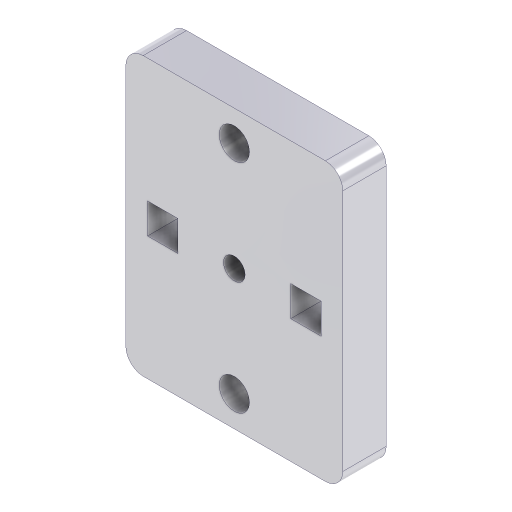
# Autodesk Inventor part: I Rückwand Adapter
Saved by Autodesk Inventor 2023 (Build 270158000, 158)
## iProperties
Created: 2022-09-18
Part Number: I Rückwand Adapter
Material: PBT-Kunststoff
Document SubType Name: Modeling
Designer: musati
Density: 1.31 g/cm^3
Appearance: Opal
Author: musati
Autodesk Inventor part; units mm, degrees
ref_plane "YZ Plane" through (0, 0, 0) normal (1, 0, 0) x (0, 1, 0)
ref_plane "XZ Plane" through (0, 0, 0) normal (0, 1, 0) x (-1, 0, 0)
ref_plane "XY Plane" through (0, 0, 0) normal (0, 0, 1) x (1, 0, 0)
sketch "Skizze1" plane through (0, 0, 0) normal (0, 0, 1) x (1, 0, 0)
  line L0 (-18.0799, 0) -> (18.0799, 0) projected
  line L1 (0, -22.9799) -> (0, 22.9799) projected
  line L2 (-10.5, -16) -> (10.5, -16)
  line L3 (12.5, -14) -> (12.5, 14)
  line L4 (10.5, 16) -> (-10.5, 16)
  line L5 (-12.5, 14) -> (-12.5, -14)
  line L6 (-12.5, -16) -> (12.5, 16) construction
  line L7 (12.5, -16) -> (-12.5, 16) construction
  arc A0 (-10.5, 16) -> (-12.5, 14) centre (-10.5, 14) ccw
  arc A1 (-12.5, -14) -> (-10.5, -16) centre (-10.5, -14) ccw
  arc A2 (10.5, -16) -> (12.5, -14) centre (10.5, -14) ccw
  arc A3 (12.5, 14) -> (10.5, 16) centre (10.5, 14) ccw
  point P0 (0, 0)
  dimension "d0" = 25
  dimension "d1" = 32
  dimension "d2" = 2
  constraints: 12 end point, 8 point on circle, 8 point on line, 8 tangent, 4 centre point, 3 equal radius, 2 midpoint, 2 parallel, 1 horizontal, 1 perpendicular
  measures "d0" distance of L7.end L6.end
  measures "d1" distance of L6.end L7.start
  measures "d2" radius of A0
extrude "Extrusion1" add sketch "Skizze1" against normal blind 5
sketch "Skizze2" plane through (0, 0, 0) normal (0, 0, 1) x (1, 0, 0)
  line L0 (12.5, -14) -> (12.5, 14) projected
  arc A0 (12.5, 14) -> (10.5, 16) centre (10.5, 14) ccw projected
  line L1 (10.5, 16) -> (-10.5, 16) projected
  arc A1 (-10.5, 16) -> (-12.5, 14) centre (-10.5, 14) ccw projected
  line L2 (-12.5, 14) -> (-12.5, -14) projected
  arc A2 (-12.5, -14) -> (-10.5, -16) centre (-10.5, -14) ccw projected
  line L3 (-10.5, -16) -> (10.5, -16) projected
  arc A3 (10.5, -16) -> (12.5, -14) centre (10.5, -14) ccw projected
  line L4 (-18.0799, 0) -> (18.0799, 0) projected
  line L5 (0, -22.9799) -> (0, 22.9799) projected
  circle A4 centre (0, 12.5) radius 1.75
  circle A5 centre (0, -12.5) radius 1.75
  point P0 (0, 0)
  dimension "d5" = 3.5
  dimension "d6" = 3.5
  dimension "d7" = 25
  dimension "d8" = 3.5
  constraints: 2 centre point, 2 point on line
  measures "d5" diameter of A4
  measures "d6" diameter of A5
  measures "d7" distance of A5.centre A4.centre
  measures "d8" distance from line of A5.centre L3
extrude "Extrusion2" cut sketch "Skizze2" against normal blind 5 contours A5 L5 | L5 A5 | A4 L5 | L5 A4
sketch "Skizze3" plane through (0, 0, 0) normal (0, 0, 1) x (1, 0, 0)
  circle A0 centre (0, -12.5) radius 1.75 projected
  circle A1 centre (0, 12.5) radius 1.75 projected
  line L0 (12.5, -14) -> (12.5, 14) projected
  arc A2 (12.5, 14) -> (10.5, 16) centre (10.5, 14) ccw projected
  line L1 (10.5, 16) -> (-10.5, 16) projected
  arc A3 (-10.5, 16) -> (-12.5, 14) centre (-10.5, 14) ccw projected
  line L2 (-12.5, 14) -> (-12.5, -14) projected
  arc A4 (-12.5, -14) -> (-10.5, -16) centre (-10.5, -14) ccw projected
  line L3 (-10.5, -16) -> (10.5, -16) projected
  arc A5 (10.5, -16) -> (12.5, -14) centre (10.5, -14) ccw projected
  line L4 (-18.0799, 0) -> (18.0799, 0) projected
  line L5 (0, -22.9799) -> (0, 22.9799) projected
  line L6 (-10, 1.75) -> (-6.5, 1.75)
  line L7 (-6.5, 1.75) -> (-6.5, -1.75)
  line L8 (-6.5, -1.75) -> (-10, -1.75)
  line L9 (-10, -1.75) -> (-10, 1.75)
  line L10 (6.5, 1.75) -> (10, 1.75)
  line L11 (10, 1.75) -> (10, -1.75)
  line L12 (10, -1.75) -> (6.5, -1.75)
  line L13 (6.5, -1.75) -> (6.5, 1.75)
  point P0 (0, 0)
  dimension "d11" = 3.5
  dimension "d12" = 3.5
  dimension "d13" = 3.5
  dimension "d14" = 3.5
  dimension "d15" = 13
  constraints: 16 end point, 4 parallel, 2 horizontal, 2 perpendicular, 1 point on line, 2 other
  measures "d11" distance of L7.end L8.end
  measures "d12" distance of L6.end L7.end
  measures "d13" distance of L11.end L12.end
  measures "d14" distance of L10.end L11.end
  measures "d15" distance between parallel lines of L13 L7
extrude "Extrusion3" cut sketch "Skizze3" against normal blind 5 contours L7 L8 L9 L4 | L4 L9 L6 L7 | L13 L10 L11 L4 | L4 L11 L12 L13
sketch "Skizze4" plane through (0, 0, 0) normal (0, 0, 1) x (1, 0, 0)
  line L0 (6.5, 1.75) -> (10, 1.75) projected
  line L1 (10, 1.75) -> (10, -1.75) projected
  line L2 (10, -1.75) -> (6.5, -1.75) projected
  line L3 (6.5, -1.75) -> (6.5, 1.75) projected
  line L4 (-10, 1.75) -> (-6.5, 1.75) projected
  line L5 (-6.5, 1.75) -> (-6.5, -1.75) projected
  line L6 (-6.5, -1.75) -> (-10, -1.75) projected
  line L7 (-10, -1.75) -> (-10, 1.75) projected
  circle A0 centre (0, -12.5) radius 1.75 projected
  circle A1 centre (0, 12.5) radius 1.75 projected
  line L8 (12.5, -14) -> (12.5, 14) projected
  arc A2 (12.5, 14) -> (10.5, 16) centre (10.5, 14) ccw projected
  line L9 (10.5, 16) -> (-10.5, 16) projected
  arc A3 (-10.5, 16) -> (-12.5, 14) centre (-10.5, 14) ccw projected
  line L10 (-12.5, 14) -> (-12.5, -14) projected
  arc A4 (-12.5, -14) -> (-10.5, -16) centre (-10.5, -14) ccw projected
  line L11 (-10.5, -16) -> (10.5, -16) projected
  arc A5 (10.5, -16) -> (12.5, -14) centre (10.5, -14) ccw projected
  line L12 (-18.0799, 0) -> (18.0799, 0) projected
  line L13 (0, -22.9799) -> (0, 22.9799) projected
  circle A6 centre (0, 0) radius 1.25
  dimension "d18" = 2.5
  constraints: 1 centre point, 1 coincident
  measures "d18" diameter of A6
extrude "Extrusion4" cut sketch "Skizze4" against normal blind 5 contours A6 L13 L12 | L12 L13 A6 | L13 A6 L12 | L12 A6 L13
